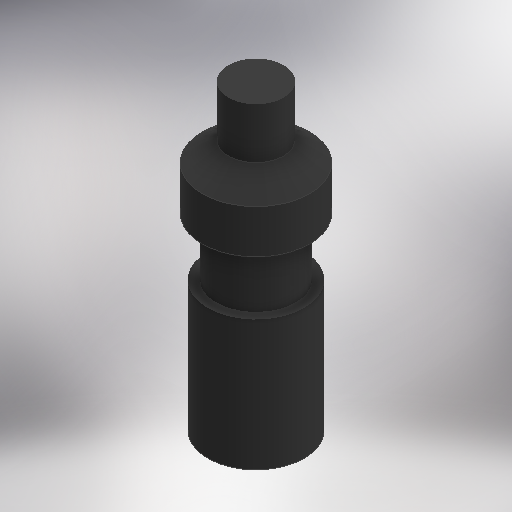
# Autodesk Inventor part: travaInternaRoda
Saved by Autodesk Inventor 2025.3 (Build 293356000, 356)
## iProperties
Created: 2026-09-17
Part Number: travaInternaRoda
Material: Genérico
Document SubType Name: Modeling
Designer: user
Density: 1 g/cm^3
Appearance: Padrão
Author: user
Autodesk Inventor part; units mm, degrees
ref_plane "YZ Plane" through (0, 0, 0) normal (1, 0, 0) x (0, 1, 0)
ref_plane "XZ Plane" through (0, 0, 0) normal (0, 1, 0) x (-1, 0, 0)
ref_plane "XY Plane" through (0, 0, 0) normal (0, 0, 1) x (1, 0, 0)
sketch "Esboço1" plane through (0, 0, 0) normal (0, 0, 1) x (1, 0, 0)
  line L0 (0, 0) -> (0, 11)
  line L1 (0, 5) -> (-10.2862, 5) construction
  line L2 (0, 9.05) -> (6.4587, 9.05) construction
  line L3 (3.2294, 11) -> (3.2294, 8.5) construction
  line L4 (1.95, 8.4353) -> (1, 9.1471)
  line L5 (1.95, 6.85) -> (1.95, 8.4353)
  line L6 (1.45, 6.85) -> (1.95, 6.85)
  line L7 (1.45, 6.85) -> (1.45, 4.75)
  line L8 (0, 4.75) -> (6.1218, 4.75) construction
  line L9 (1.75, 4.75) -> (1.75, 0)
  line L10 (1.75, 4.75) -> (1.45, 4.75)
  line L11 (0, 11) -> (1, 11)
  line L12 (1, 11) -> (1, 9.1471)
  line L13 (0, 0) -> (1.75, 0)
  point P0 (0, 0)
  dimension "d17" = 1
  dimension "d24" = 1.95
  dimension "d25" = 1.75
  dimension "d26" = 2.1
  dimension "d27" = 1.45
  constraints: 28 end point, 5 point on line, 3 perpendicular, 2 vertical, 1 horizontal
  measures "d17" distance of L0.end L11.end
  measures "d24" distance between parallel lines of L0 L5
  measures "d25" distance between parallel lines of L9 L0
  measures "d26" distance of L6.start L7.end
  measures "d27" distance between parallel lines of L0 L7
revolve "Revolução1" add sketch "Esboço1" angle 360 about axis through (0, 0, 0) along (0, 1, 0)
